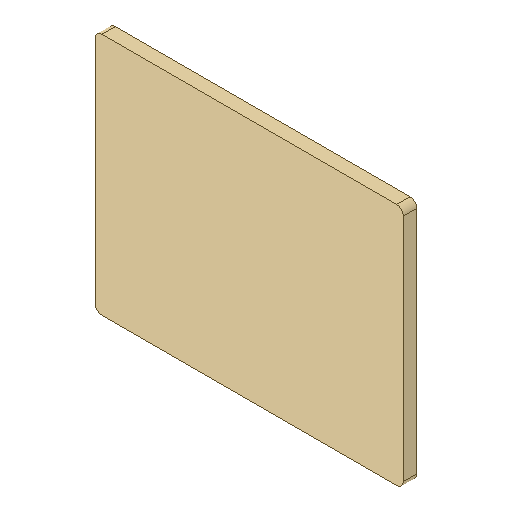
# Autodesk Inventor part: 3DP_PLA_Front_filter_mesh
Saved by Autodesk Inventor 2025 (Build 290162010, 162A)
## iProperties
Created: 2020-03-29
Part Number: 3DP_PLA_Front_filter_mesh
Material: Generic
Document SubType Name: Modeling
Designer: Andrzej
Density: 1 g/cm^3
Appearance: Wheat
Author: Andrzej
Autodesk Inventor part; units mm, degrees
ref_plane "YZ Plane" through (0, 0, 0) normal (1, 0, 0) x (0, 1, 0)
ref_plane "XZ Plane" through (0, 0, 0) normal (0, 1, 0) x (-1, 0, 0)
ref_plane "XY Plane" through (0, 0, 0) normal (0, 0, 1) x (1, 0, 0)
sketch "Sketch1" plane through (0, 0, 0) normal (0, 0, 1) x (1, 0, 0)
  line L0 (-64.9326, 48.6525) -> (73.0674, 48.6525)
  line L1 (73.0674, 48.6525) -> (73.0674, -60.3475)
  line L2 (73.0674, -60.3475) -> (-64.9326, -60.3475)
  line L3 (-64.9326, -60.3475) -> (-64.9326, 48.6525)
  point P0 (0, 0)
  dimension "d0" = 138
  dimension "d1" = 109
  constraints: 8 end point, 2 parallel, 1 horizontal, 1 perpendicular
  measures "d0" distance of L1.end L2.end
  measures "d1" distance of L0.end L1.end
extrude "Extrusion1" add sketch "Sketch1" along normal blind 6
fillet "Fillet1" radius 3 4 edges at (73.0674, 48.6525, 3) (-64.9326, 48.6525, 3) (73.0674, -60.3475, 3) (-64.9326, -60.3475, 3)
body "Solid1"
